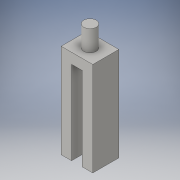
# Autodesk Inventor part: Control Board Ring Slot Holder
Saved by Autodesk Inventor 2016 (Build 200138000, 138)
## iProperties
Created: 2017-10-23
Part Number: Control Board Ring Slot Holder
Material: Generic
Document SubType Name: Modeling
Designer: Student
Density: 1 g/cm^3
Appearance: Default
Author: Student
Autodesk Inventor part; units mm, degrees
ref_plane "YZ Plane" through (0, 0, 0) normal (1, 0, 0) x (0, 1, 0)
ref_plane "XZ Plane" through (0, 0, 0) normal (0, 1, 0) x (-1, 0, 0)
ref_plane "XY Plane" through (0, 0, 0) normal (0, 0, 1) x (1, 0, 0)
sketch "Sketch1" plane through (0, 0, 0) normal (0, 1, 0) x (-1, 0, 0)
  line L0 (3.2881, 3.6219) -> (-4.4081, 3.6219)
  line L1 (-4.4081, 3.6219) -> (-4.4081, -2.7281)
  line L2 (-4.4081, -2.7281) -> (3.2881, -2.7281)
  line L3 (3.2881, -2.7281) -> (3.2881, 3.6219)
  point P0 (0, 0)
  dimension "d0" = 7.6962
  dimension "d1" = 6.35
  constraints: 8 end point, 2 parallel, 1 horizontal, 1 perpendicular
  measures "d0" distance of L1.end L2.end
  measures "d1" distance of L2.end L0.start
extrude "Extrusion1" add sketch "Sketch1" along normal blind 2.54
sketch "Sketch2" plane through (0, 2.54, 0) normal (0, 1, 0) x (1, 0, 0)
  circle A0 centre (0.56, -0.4469) radius 1.5
  line L0 (4.4081, 2.7281) -> (-3.2881, 2.7281) projected
  line L1 (-3.2881, 2.7281) -> (-3.2881, -3.6219) projected
  point P0 (0, 0)
  point P1 (0.56, 2.7281)
  point P2 (-3.2881, -0.4469)
  dimension "d4" = 3
  constraints: 2 midpoint, 1 centre point, 1 horizontal alignment, 1 vertical alignment
  measures "d4" diameter of A0
extrude "Extrusion2" add sketch "Sketch2" along normal blind 5.08
sketch "Sketch3" plane through (0, 0, 0) normal (0, -1, 0) x (1, 0, 0)
  line L0 (-3.2881, -2.7281) -> (-3.2881, 3.6219) projected
  line L1 (-3.2881, -2.7281) -> (-0.7481, -2.7281)
  line L2 (-0.7481, -2.7281) -> (-0.7481, 3.6219)
  line L3 (-0.7481, 3.6219) -> (-3.2881, 3.6219)
  line L4 (-3.2881, 3.6219) -> (-3.2881, -2.7281)
  line L5 (4.4081, -2.7281) -> (1.8681, -2.7281)
  line L6 (1.8681, -2.7281) -> (1.8681, 3.6219)
  line L7 (1.8681, 3.6219) -> (4.4081, 3.6219)
  line L8 (4.4081, 3.6219) -> (4.4081, -2.7281)
  point P0 (0, 0)
  dimension "d7" = 2.54
  dimension "d8" = 2.54
  dimension "d9" = 2.6162
  constraints: 16 end point, 4 parallel, 2 horizontal, 2 perpendicular
  measures "d7" distance of L2.end L3.end
  measures "d8" distance of L6.end L7.end
  measures "d9" distance between parallel lines of L6 L2
extrude "Extrusion3" add sketch "Sketch3" along normal blind 20.32
equation "\"d8\" = d7"
body "Solid1"
